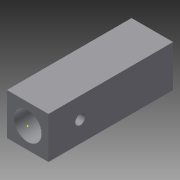
# Autodesk Inventor part: MotorBarMount
Saved by Autodesk Inventor 2015 (Build 190159000, 159)
## iProperties
Created: 2016-05-03
Part Number: MotorBarMount
Material: Generic
Document SubType Name: Modeling
Designer: Hatch
Density: 1 g/cm^3
Appearance: Default
Author: Hatch
Autodesk Inventor part; units mm, degrees
ref_plane "YZ Plane" through (0, 0, 0) normal (1, 0, 0) x (0, 1, 0)
ref_plane "XZ Plane" through (0, 0, 0) normal (0, 1, 0) x (-1, 0, 0)
ref_plane "XY Plane" through (0, 0, 0) normal (0, 0, 1) x (1, 0, 0)
sketch "Sketch1" plane through (0, 0, 0) normal (0, 1, 0) x (-1, 0, 0)
  circle A0 centre (0, 0) radius 5
  circle A1 centre (0, 0) radius 7.5
  dimension "d0" = 10
  dimension "d1" = 15
  constraints: 2 centre point, 2 coincident
  measures "d0" diameter of A0
  measures "d1" diameter of A1
extrude "Extrusion1" add sketch "Sketch1" along normal blind 25
sketch "Sketch2" plane through (0, 25, 0) normal (0, 1, 0) x (1, 0, 0)
  circle A0 centre (0, 0) radius 5
  constraints: 1 centre point, 1 coincident
extrude "Extrusion2" add sketch "Sketch2" along normal blind 20
sketch "Sketch3" plane through (0, 25, 0) normal (0, -1, 0) x (1, 0, 0)
  circle A0 centre (0, 0) radius 5
  constraints: 1 centre point, 1 coincident
extrude "Extrusion3" add sketch "Sketch3" along normal blind 5
sketch "Sketch4" plane through (0, 45, 0) normal (0, 1, 0) x (1, 0, 0)
  circle A0 centre (0, 0) radius 2.125
  dimension "d8" = 4.25
  constraints: 1 centre point, 1 coincident
  measures "d8" diameter of A0
extrude "Extrusion4" cut sketch "Sketch4" against normal blind 15
sketch "Sketch5" plane through (0, 45, 0) normal (0, 1, 0) x (1, 0, 0)
  circle A0 centre (0, 0) radius 2.125 projected
  line L0 (2.125, 0) -> (-1.125, 0)
  line L1 (-1.0625, 1.8403) -> (-1.0625, -1.8403)
  arc A1 (-1.0625, 1.8403) -> (-1.0625, -1.8403) centre (0, 0) ccw
  dimension "d11" = 3.25
  constraints: 5 point on circle, 4 end point, 1 centre point, 1 concentric, 1 horizontal, 1 perpendicular
  measures "d11" distance of L0.start L0.end
extrude "Extrusion5" add sketch "Sketch5" against normal blind 15 contours L1 A0
sketch "Sketch6" plane through (-1.0625, 45, 1.8403) normal (1, 0, 0) x (0, 0, -1)
  line L0 (3.6806, 0) -> (0, 0)
  line L1 (0, -15) -> (0, 0) projected
  line L2 (6.8403, 0) -> (-3.1597, 0) projected
  line L3 (1.8403, 0) -> (1.8403, -8)
  circle A0 centre (1.8403, -8) radius 2
  point P0 (1.8403, -45)
  dimension "d14" = 8
  dimension "d15" = 4
  constraints: 4 end point, 1 centre point, 1 coincident, 1 midpoint, 1 perpendicular, 1 vertical
  measures "d14" distance of L3.start L3.end
  measures "d15" diameter of A0
extrude "Extrusion6" cut sketch "Sketch6" against normal through all contours A0 L1 | L1 A0
sketch "Sketch7" plane through (0, 0, 0) normal (0, -1, 0) x (1, 0, 0)
  line L0 (-7.5, -7.5) -> (7.5, -7.5)
  line L1 (7.5, -7.5) -> (7.5, 7.5)
  line L2 (7.5, 7.5) -> (-7.5, 7.5)
  line L3 (-7.5, 7.5) -> (-7.5, -7.5)
  arc A0 (-1.0625, -1.8403) -> (-1.0625, 1.8403) centre (0, 0) ccw projected
  line L4 (-7.5, -7.5) -> (7.5, 7.5) construction
  line L5 (7.5, -7.5) -> (-7.5, 7.5) construction
  circle A1 centre (0, 0) radius 7.5
  constraints: 12 end point, 2 midpoint, 2 parallel, 1 centre point, 1 coincident, 1 horizontal, 1 perpendicular
extrude "Extrusion7" add sketch "Sketch7" against normal blind 25 contours L3 A1 L0 | A1 L1 L0 | L3 L2 A1 | A1 L2 L1
sketch "Sketch8" plane through (7.5, 0, 7.5) normal (1, 0, 0) x (0, 0, -1)
  circle A0 centre (7.5, 11.4586) radius 1.75
  point P0 (7.5, 0)
  dimension "d20" = 3.5
  constraints: 1 centre point
  measures "d20" diameter of A0
extrude "Extrusion8" cut sketch "Sketch8" against normal blind 3.5
sketch "Sketch9" plane through (0, 25, 0) normal (0, 1, 0) x (1, 0, 0)
  line L0 (7.5, -7.5) -> (-7.5, -7.5)
  line L1 (-7.5, -7.5) -> (-7.5, 7.5)
  line L2 (-7.5, 7.5) -> (7.5, 7.5)
  line L3 (7.5, 7.5) -> (7.5, -7.5)
  line L4 (7.5, -7.5) -> (-7.5, 7.5) construction
  line L5 (-7.5, -7.5) -> (7.5, 7.5) construction
  circle A0 centre (0, 0) radius 5
  constraints: 12 end point, 2 midpoint, 2 parallel, 1 centre point, 1 coincident, 1 horizontal, 1 perpendicular
extrude "Extrusion9" add sketch "Sketch9" along normal blind 20
sketch "Sketch12" plane through (-7.5, 0, -7.5) normal (-1, 0, 0) x (0, 0, 1)
  arc A0 (5.6597, 37.7831) -> (5.6597, 36.2169) centre (7.5, 37) ccw projected
  circle A1 centre (7.5, 37) radius 2
  point P0 (7.5, 0)
  constraints: 1 centre point, 1 coincident
extrude "Extrusion10" cut sketch "Sketch12" against normal blind 8
sketch "Sketch13" plane through (0, 0, 0) normal (0, -1, 0) x (1, 0, 0)
  point P0 (0, 0)
equation "\"d21\" = d20"
body "Solid1"
